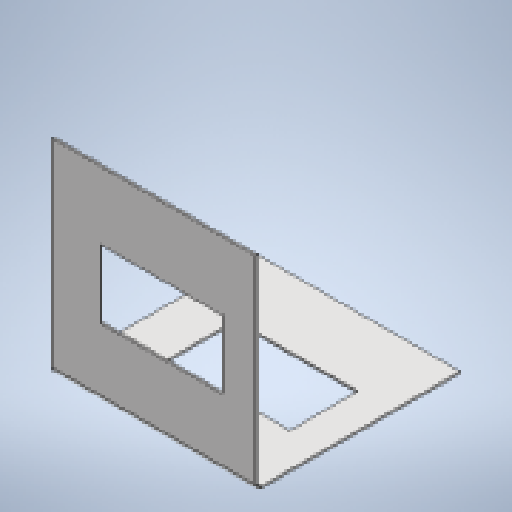
# Autodesk Inventor part: TKS 3004 BOTTOM DS box wall 1
Saved by Autodesk Inventor 2025 (Build 290162010, 162A)
## iProperties
Created: 2024-12-09
Part Number: TKS 3004 BOTTOM DS box wall 1
Material: Stainless Steel
Document SubType Name: Sheet Metal
Designer: user
Mass: 3269.02 g
Surface Area: 1007.63 cm^2
Volume: 408.627 cm^3
Density: 8 g/cm^3
Flat Pattern Width: 59.3927 cm
Flat Pattern Length: 30 cm
Flat Pattern Area: 1781.78 cm^2
Sheet Metal Rule: AISI304 3mm Die 32
Sheet Metal Width: 593,927 mm
Sheet Metal Length: 300,000 mm
Sheet Metal Area: 178178,230 mm^2
Appearance: Default
Author: user
Autodesk Inventor part; units mm, degrees
ref_plane "YZ Plane" through (0, 0, 0) normal (1, 0, 0) x (0, 1, 0)
ref_plane "XZ Plane" through (0, 0, 0) normal (0, 1, 0) x (-1, 0, 0)
ref_plane "XY Plane" through (0, 0, 0) normal (0, 0, 1) x (1, 0, 0)
sketch "Sketch1" plane through (0, 0, 0) normal (0, 0, 1) x (1, 0, 0)
  line L0 (150, 150) -> (-150, 150)
  line L1 (-150, 150) -> (-150, -150)
  line L2 (-150, -150) -> (150, -150)
  line L3 (150, -150) -> (150, 150)
  line L4 (150, 150) -> (-150, -150) construction
  line L5 (-150, 150) -> (150, -150) construction
  line L6 (100, 50) -> (-80, 50)
  line L7 (-80, 50) -> (-80, -50)
  line L8 (-80, -50) -> (100, -50)
  line L9 (100, -50) -> (100, 50)
  line L10 (100, 50) -> (-80, -50) construction
  line L11 (-80, 50) -> (100, -50) construction
  point P0 (0, 0)
  point P1 (0, 0)
  point P2 (10, 0)
  point P3 (100, 0)
  point P4 (150, 0)
  dimension "d32" = 300
  dimension "d33" = 300
  dimension "d34" = 180
  dimension "d35" = 100
  dimension "d51" = 50
  measures "d32" distance of L2.end L0.start
  measures "d33" distance of L1.end L2.end
  measures "d34" distance of L7.end L8.end
  measures "d35" distance of L8.end L6.start
  measures "d51" distance between parallel lines of L9 L3
extrude "Plate1" add sketch "Sketch1" along normal blind 3
sketch "Sketch6" plane through (150, -147, 0) normal (0, -1, 0) x (1, 0, 0)
  line L0 (-300, 0) -> (0, 0)
  line L1 (0, 0) -> (0, 300)
  line L2 (0, 300) -> (-300, 300)
  line L3 (-300, 300) -> (-300, 0)
  constraints: 6 end point, 1 horizontal, 1 perpendicular, 1 vertical
edge flange "Flange2" height 300 angle 90 thickness 3 bend radius 5 thickness toward (0, -1, 0) relief round relief width 3 relief depth 1.5 edges at (0, -150, 3) wall of the first edge with corners at (-150, -147, 0) (150, -147, 0) (150, -147, 300) (-150, -147, 300)
bend "Bend2"
corner "Corner2"
sketch "Sketch7" plane through (-150, -147, 300) normal (0, 1, 0) x (1, 0, 0)
  line L0 (0, 292) -> (300, 292) construction
  line L1 (300, 0) -> (300, 292) projected
  line L2 (0, 0) -> (300, 0) construction
  line L3 (0, 292) -> (0, 0) construction
  line L4 (70, 100) -> (250, 100)
  line L5 (250, 100) -> (250, 200)
  line L6 (250, 200) -> (70, 200)
  line L7 (70, 200) -> (70, 100)
  line L8 (70, 100) -> (250, 200) construction
  line L9 (250, 100) -> (70, 200) construction
  line L10 (300, 300) -> (0, 300) projected
  line L11 (300, 300) -> (0, 300) projected
  line L12 (70, 300) -> (250, 300) projected
  line L13 (250, 300) -> (70, 300) projected
  line L14 (300, 150) -> (0, 150) construction
  line L15 (261.5016, 150) -> (261.5016, 0) construction
  line L16 (261.5016, 300) -> (261.5016, 150) construction
  point P0 (150, 300)
  point P1 (160, 150)
  dimension "d46" = 180
  dimension "d47" = 100
  dimension "d52" = 50
  constraints: 18 end point, 7 point on line, 3 equal length, 3 perpendicular, 2 midpoint, 1 collinear, 1 horizontal
  measures "d46" distance of L6.end L5.end
  measures "d47" distance of L5.end L4.end
  measures "d52" distance between parallel lines of L5 L1
extrude "Cut2" cut sketch "Sketch7" against normal blind 3
equation "\"d46\" = d34"
equation "\"d47\" = d35"
equation "\"d52\" = d51"
equation "\"d49\" = Thickness"
equation "\"d2\" = Thickness"
equation "\"d36\" = BendReliefWidth"
equation "\"d37\" = BendReliefDepth"
equation "\"d38\" = MinimumRemnant"
equation "\"d39\" = TransitionRadius"
equation "\"d42\" = BendRadius"
equation "\"d43\" = CornerReliefSize"
equation "\"d44\" = GapSize"
equation "\"d45\" = JacobiRadiusSize"
equation "\"BendReliefWidth\" = Thickness"
equation "\"BendReliefDepth\" = 0.5 * Thickness"
equation "\"CornerReliefSize\" = 4 * Thickness"
equation "\"MinimumRemnant\" = 2 * Thickness"
equation "\"TransitionRadius\" = BendRadius"
equation "\"JacobiRadiusSize\" = BendRadius"
equation "\"GapSize\" = Thickness"
equation "\"Thickness\" = 3"
equation "\"BendRadius\" = 5"
body "Solid1"
